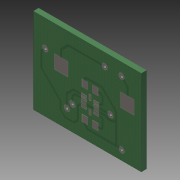
# Autodesk Inventor part: Health_module_contactBoard
Saved by Autodesk Inventor 2013 (Build 170138000, 138)
## iProperties
Created: 2015-07-04
Part Number: Health_module_contactBoard
Material: Ogólny
Document SubType Name: Modeling
Designer: terg
Density: 1 g/cm^3
Author: terg
Autodesk Inventor part; units mm, degrees
ref_plane "YZ Plane" through (0, 0, 0) normal (1, 0, 0) x (0, 1, 0)
ref_plane "XZ Plane" through (0, 0, 0) normal (0, 1, 0) x (-1, 0, 0)
ref_plane "XY Plane" through (0, 0, 0) normal (0, 0, 1) x (1, 0, 0)
sketch "Szkic1" plane through (0, 0, 0) normal (0, 1, 0) x (-1, 0, 0)
  line L0 (0, 0) -> (16.4, 0)
  line L1 (16.4, 0) -> (16.4, 13)
  line L2 (16.4, 13) -> (0, 13)
  line L3 (0, 13) -> (0, 0)
  dimension "d0" = 16.4
  dimension "d1" = 13
  constraints: 8 end point, 2 parallel, 1 horizontal, 1 perpendicular
  measures "d0" distance of L2.end L1.end
  measures "d1" distance of L1.end L0.end
extrude "Wyciągnięcie proste1" add sketch "Szkic1" along normal blind 0.8
sketch "Szkic2" plane through (0, 0.8, 0) normal (0, 1, 0) x (1, 0, 0)
  line L0 (0, 0) -> (-16.4, 0) projected
  line L1 (-16.4, 0) -> (-16.4, -13) projected
  line L2 (-16.4, -13) -> (0, -13) projected
  line L3 (0, -13) -> (0, 0) projected
  line L4 (-16.4015, 0) -> (0.0015, 0) construction
  line L5 (0.0015, 0) -> (0.0015, -13) construction
  line L6 (0.0015, -13) -> (-16.4015, -13) construction
  line L7 (-16.4015, -13) -> (-16.4015, 0) construction
  dimension "d9" = 0
  dimension "d10" = -0.0015
  dimension "d11" = 0
  dimension "d12" = -0.0015
  constraints: 2 other
  measures "d9" distance between parallel lines of L0 L4
  measures "d10" distance between parallel lines of L3 L5
  measures "d11" distance between parallel lines of L2 L6
  measures "d12" distance between parallel lines of L1 L7
decal "Pokrycie bitmapą1"
sketch "Szkic3" plane through (0, 0, 0) normal (0, -1, 0) x (1, 0, 0)
  line L0 (0, 0) -> (-16.4, 0) projected
  line L1 (0, 13) -> (0, 0) projected
  line L2 (-16.4, 13) -> (0, 13) projected
  line L3 (-16.4, 0) -> (-16.4, 13) projected
  line L4 (0.0015, 0) -> (-16.4015, 0) construction
  line L5 (-16.4015, 0) -> (-16.4015, 13) construction
  line L6 (-16.4015, 13) -> (0.0015, 13) construction
  line L7 (0.0015, 13) -> (0.0015, 0) construction
  dimension "d23" = 0
  dimension "d24" = -0.0015
  dimension "d25" = 0
  dimension "d26" = -0.0015
  constraints: 2 other
  measures "d23" distance between parallel lines of L0 L4
  measures "d24" distance between parallel lines of L3 L5
  measures "d25" distance between parallel lines of L2 L6
  measures "d26" distance between parallel lines of L1 L7
decal "Pokrycie bitmapą2"
sketch "Szkic4" plane through (0, 0, 0) normal (0, -1, 0) x (1, 0, 0)
  point P0 (-14.594, 8.979)
  point P1 (-5.5831, 11.1285)
  point P2 (-3.0054, 11.0897)
  point P3 (-3.0054, 1.4497)
  point P4 (-4.699, 5.2329)
  point P5 (-10.4866, 3.7398)
  point P6 (-11.3289, 2.754)
hole "Otwór1" at (-14.594, 0, 8.979) at (-5.5831, 0, 11.1285) at (-3.0054, 0, 11.0897) at (-3.0054, 0, 1.4497) at (-4.699, 0, 5.2329) at (-10.4866, 0, 3.7398) at (-11.3289, 0, 2.754) direction (0, 1, 0) diameter 0.4 depth 8
equation "\"d10\" = d12"
equation "\"d24\" = d26"
